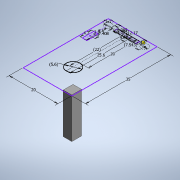
# Autodesk Inventor part: Electromagnet Measurements
Saved by Autodesk Inventor 2020.5 (Build 245400000, 400)
## iProperties
Created: 2023-03-23
Part Number: Electromagnet Measurements
Material: Generic
Document SubType Name: Modeling
Designer: Wes
Density: 1 g/cm^3
Appearance: Default
Author: Wes
Autodesk Inventor part; units mm, degrees
ref_plane "YZ Plane" through (0, 0, 0) normal (1, 0, 0) x (0, 1, 0)
ref_plane "XZ Plane" through (0, 0, 0) normal (0, 1, 0) x (-1, 0, 0)
ref_plane "XY Plane" through (0, 0, 0) normal (0, 0, 1) x (1, 0, 0)
sketch "Sketch1" plane through (0, 0, 0) normal (0, 0, 1) x (1, 0, 0)
  line L0 (0, 0) -> (0, 18) construction
  line L1 (0, 9) -> (0, 2.915) construction
  line L2 (0, 9) -> (0, 15.085) construction
  line L3 (0, 2.915) -> (0, 0) construction
  line L4 (0, 15.085) -> (0, 18) construction
  circle A0 centre (0, 1.4575) radius 1.4575 construction
  circle A1 centre (0, 16.5425) radius 1.4575 construction
  line L5 (0, 9) -> (0, 13.525) construction
  line L6 (0, 9) -> (0, 4.475) construction
  line L7 (-0.8, 4.475) -> (0.8, 4.475)
  line L8 (0.8, 4.475) -> (0.8, 13.525)
  line L9 (0.8, 13.525) -> (-0.8, 13.525)
  line L10 (-0.8, 13.525) -> (-0.8, 4.475)
  line L11 (-0.8, 4.475) -> (0.8, 13.525) construction
  line L12 (0.8, 4.475) -> (-0.8, 13.525) construction
  line L13 (1.4575, 1.4575) -> (9.7575, 1.4575) construction
  line L14 (1.4575, 1.4575) -> (5.0575, 1.4575) construction
  line L15 (5.0575, 1.4575) -> (9.7575, 1.4575) construction
  line L16 (9.7575, 0.5075) -> (5.0575, 0.5075)
  line L17 (5.0575, 0.5075) -> (5.0575, 2.4075)
  line L18 (5.0575, 2.4075) -> (9.7575, 2.4075)
  line L19 (9.7575, 2.4075) -> (9.7575, 0.5075)
  line L20 (9.7575, 0.5075) -> (5.0575, 2.4075) construction
  line L21 (5.0575, 0.5075) -> (9.7575, 2.4075) construction
  line L22 (-0.8, 9) -> (24.8, 9) construction
  line L23 (-0.8, 9) -> (19.2, 9) construction
  line L24 (19.2, 9) -> (24.8, 9) construction
  circle A2 centre (22, 9) radius 2.8
  line L25 (-1.4575, 1.4575) -> (-2.4575, 1.4575) construction
  line L26 (0, 0) -> (0, -1) construction
  line L27 (-2.4575, -1) -> (32.5425, -1)
  line L28 (32.5425, -1) -> (32.5425, 19)
  line L29 (32.5425, 19) -> (-2.4575, 19)
  line L30 (-2.4575, 19) -> (-2.4575, -1)
  line L31 (0, 1.4575) -> (7.408, 1.4577) construction
  line L32 (22, 9) -> (0, 9) construction
  point P0 (7.4075, 1.4575)
  dimension "d23" = 5.6
  dimension "d0" = 18
  dimension "d1" = 6.085
  dimension "d3" = 12.17
  dimension "d5" = 4.525
  dimension "d6" = 9.05
  dimension "d7" = 1.6
  dimension "d8" = 8.3
  dimension "d9" = 3.6
  dimension "d10" = 1.9
  dimension "d11" = 25.6
  dimension "d12" = 20
  dimension "d13" = 1
  dimension "d14" = 1
  dimension "d15" = 35
  dimension "d16" = 20
  dimension "d19" = 7.5425
  dimension "d20" = 7.408
  dimension "d21" = 4.7
  dimension "d22" = 22
  constraints: 66 end point, 10 midpoint, 7 horizontal, 7 point on line, 6 parallel, 4 collinear, 3 perpendicular, 3 point on circle, 2 vertical, 1 centre point, 1 horizontal alignment, 1 vertical alignment, 4 other
  measures "d0" distance of L0.start L0.end
  measures "d1" distance of L1.start L1.end
  measures "d3" distance of L2.end L1.end
  measures "d5" distance of L1.start L6.end
  measures "d6" distance of L5.end L6.end
  measures "d7" distance of L9.end L8.end
  measures "d8" distance of L13.start L13.end
  measures "d9" distance of L13.start L14.end
  measures "d10" distance of L16.end L17.end
  measures "d11" distance of L22.start L22.end
  measures "d12" distance of L22.start L23.end
  measures "d13" distance of L25.start L25.end
  measures "d14" distance of L0.start L26.end
  measures "d15" distance of L29.end L28.end
  measures "d16" distance of L28.end L27.end
  measures "d19" distance of point (0, 16.543) L1.start
  measures "d20" distance of L31.start L31.end
  measures "d21" distance of L16.start L16.end
  measures "d22" distance of L32.start L1.start
sketch "Sketch2" plane through (0, 0, 0) normal (0, 0, 1) x (1, 0, 0)
  line L0 (32.2063, 18.719) -> (28.2081, 18.719)
  line L1 (28.2081, 18.719) -> (28.2081, 15.2206)
  line L2 (28.2081, 15.2206) -> (32.2063, 15.2206)
  line L3 (32.2063, 15.2206) -> (32.2063, 18.719)
  point P0 (0, 0)
  constraints: 8 end point, 2 parallel, 1 horizontal, 1 perpendicular
extrude "Extrusion1" add sketch "Sketch2" against normal blind 16.6
body "Solid1"
